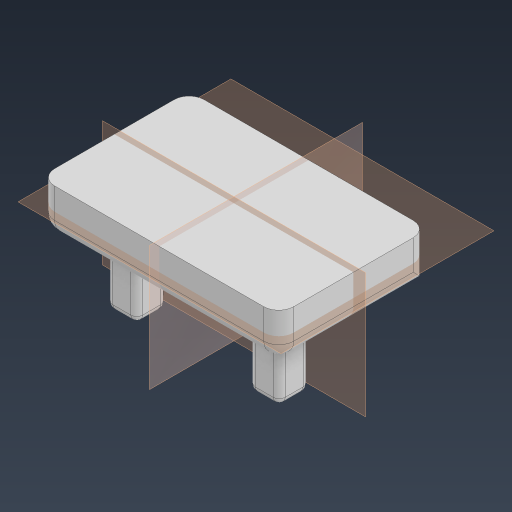
# Autodesk Inventor part: Крепление_камеры
Saved by Autodesk Inventor 2023.2 (Build 272271030, 271C)
## iProperties
Created: 2025-10-07
Part Number: Крепление_камеры
Material: Типовые
Document SubType Name: Modeling
Designer: Олег Коноваленко
Density: 1 g/cm^3
Appearance: По умолчанию
Author: Олег Коноваленко
Autodesk Inventor part; units mm, degrees
sketch "Эскиз1" plane through (0, 0, 0) normal (0, 1, 0) x (-1, 0, 0)
  line L0 (40, 25) -> (-40, 25)
  line L1 (-40, 25) -> (-40, -25)
  line L2 (-40, -25) -> (40, -25)
  line L3 (40, -25) -> (40, 25)
  line L4 (40, 25) -> (-40, -25) construction
  line L5 (-40, 25) -> (40, -25) construction
  point P0 (0, 0)
  dimension "d0" = 50
  dimension "d1" = 80
  constraints: 12 end point, 2 midpoint, 2 parallel, 1 horizontal, 1 perpendicular
  measures "d0" distance of L0.end L1.end
  measures "d1" distance of L1.end L2.end
extrude "Выдавливание1" add sketch "Эскиз1" along normal mid plane 15
sketch "Эскиз3" plane through (0, 0, 0) normal (1, 0, 0) x (0, 1, 0)
  circle A0 centre (-11.4044, -36.1632) radius 3.6
  circle A1 centre (-11.4044, -36.1632) radius 1.6
  line L0 (-7.5, -25) -> (7.5, -25) projected
  line L1 (-7.5, -25) -> (-14.2795, -33.9967)
  line L2 (7.5, -25) -> (-9.0903, -38.921)
  line L3 (-7.5, -25) -> (-7.5, 25) projected
  point P0 (0, 0)
  dimension "d6" = 3.2
  dimension "d7" = 7.2
  dimension "d11" = 40
  dimension "d29" = 127
  constraints: 4 end point, 2 centre point, 2 point on circle, 2 tangent, 1 coincident
  measures "d6" diameter of A1
  measures "d7" diameter of A0
  measures "d11" angle of L0 L2
  measures "d29" angle of L0 L1
extrude "Выдавливание2" add sketch "Эскиз3" along normal mid plane 20
sketch "Эскиз4" plane through (0, -7.5, 0) normal (0, -1, 0) x (1, 0, 0)
  line L0 (-28.825, 3.6843) -> (-28.825, 13.6843)
  line L1 (-28.825, 13.6843) -> (-18.825, 13.6843)
  line L2 (-18.825, 13.6843) -> (-18.825, 3.6843)
  line L3 (-18.825, 3.6843) -> (-28.825, 3.6843)
  line L4 (-12.825, 6.5843) -> (-17.825, 6.5843)
  line L5 (-12.825, 10.7843) -> (-17.825, 10.7843)
  line L6 (-17.825, 6.5843) -> (-17.825, 10.7843)
  point P0 (0, 0)
  dimension "d14" = 10
  dimension "d18" = 10
  dimension "d22" = 1
  dimension "d23" = 2.9
  constraints: 14 end point, 2 horizontal, 2 perpendicular, 2 vertical, 1 parallel, 4 other
  measures "d14" distance of L0.end L1.end
  measures "d18" distance of L0.start L0.end
  measures "d22" distance between parallel lines of L6 L2
  measures "d23" distance between parallel lines of L1 L5
extrude "Выдавливание3" add sketch "Эскиз4" along normal blind 23
fillet "Сопряжение1" radius 2 12 edges at (-23.825, -30.5, 13.6843) (-18.825, -30.5, 8.6843) (-23.825, -30.5, 3.6843) (-28.825, -30.5, 8.6843) (-23.825, -7.5, 3.6843) (-28.825, -7.5, 8.6843) (-18.825, -19, 3.6843) (-28.825, -19, 3.6843) (-28.825, -19, 13.6843) (-18.825, -19, 13.6843) (-23.825, -7.5, 13.6843) (-18.825, -7.5, 8.6843)
sketch "Эскиз5" plane through (-18.825, -7.5, 13.6843) normal (1, 0, 0) x (0, 0, -1)
  circle A0 centre (11.6545, -18.8946) radius 2.1 projected
  point P0 (13.6843, 7.5)
extrude "Выдавливание4" cut sketch "Эскиз5" against normal up to next
sketch "Эскиз6" plane through (0, 0, 0) normal (1, 0, 0) x (0, 1, 0)
  line L0 (-14.2795, -33.9967) -> (-7.5, -25) projected
  line L1 (7.5, -25) -> (-7.5, -25) projected
  line L2 (7.5, -25) -> (-9.0903, -38.921) projected
  arc A0 (-14.2795, -33.9967) -> (-9.0903, -38.921) centre (-11.4044, -36.1632) ccw projected
  circle A1 centre (-11.4044, -36.1632) radius 1.6 projected
  point P0 (0, 0)
extrude "Выдавливание5" cut sketch "Эскиз6" along normal mid plane 7 contours L0 L1 L2 A0 | A1
fillet "Сопряжение3" radius 5 7 edges at (-40, 0, 25) (-40, 0, -25) (40, 0, 25) (40, 0, -25) (40, -7.5, 0) (0, -7.5, 25) (-40, -7.5, 0)
mirror "Зеркальное отражение1" about plane through (0, 0, 0) normal (1, 0, 0) of "Выдавливание3", "Сопряжение1"
